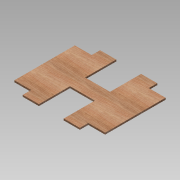
# Autodesk Inventor part: base board
Saved by Autodesk Inventor 2015 (Build 190159000, 159)
## iProperties
Created: 2015-12-17
Part Number: base board
Material: Wood (Birch)
Document SubType Name: Modeling
Designer: Daniel
Density: 0.55 g/cm^3
Appearance: Birch - Natural Polished
Author: Daniel
Autodesk Inventor part; units mm, degrees
ref_plane "YZ Plane" through (0, 0, 0) normal (1, 0, 0) x (0, 1, 0)
ref_plane "XZ Plane" through (0, 0, 0) normal (0, 1, 0) x (-1, 0, 0)
ref_plane "XY Plane" through (0, 0, 0) normal (0, 0, 1) x (1, 0, 0)
sketch "Sketch1" plane through (0, 0, 0) normal (0, 1, 0) x (-1, 0, 0)
  line L0 (0, 0) -> (685.8, 0)
  line L1 (685.8, 0) -> (685.8, -584.2)
  line L2 (685.8, -584.2) -> (0, -584.2)
  line L3 (0, -584.2) -> (0, 0)
  dimension "d0" = 685.8
  dimension "d1" = 584.2
  constraints: 8 end point, 2 parallel, 1 horizontal, 1 perpendicular
  measures "d0" distance of L0.start L0.end
  measures "d1" distance of L2.end L0.start
extrude "Extrusion1" add sketch "Sketch1" along normal blind 12.7
sketch "Sketch2" plane through (0, 12.7, 0) normal (0, 1, 0) x (1, 0, 0)
  line L0 (-436.88, 0) -> (-248.92, 0)
  line L1 (-248.92, 0) -> (-248.92, 234.95)
  line L2 (-248.92, 234.95) -> (-436.88, 234.95)
  line L3 (-436.88, 234.95) -> (-436.88, 0)
  line L4 (0, 584.2) -> (-685.8, 584.2) projected
  line L5 (-436.88, 584.2) -> (-248.92, 584.2)
  line L6 (-248.92, 584.2) -> (-248.92, 349.25)
  line L7 (-248.92, 349.25) -> (-436.88, 349.25)
  line L8 (-436.88, 349.25) -> (-436.88, 584.2)
  line L9 (-685.8, 0) -> (0, 0) projected
  line L10 (-436.88, 349.25) -> (-436.88, 234.95) construction
  line L11 (-685.8, 584.2) -> (-685.8, 0) construction
  point P0 (-342.9, 0)
  point P1 (-342.9, 0)
  point P2 (-342.9, 0)
  point P3 (-342.9, 584.2)
  point P4 (-342.9, 584.2)
  point P5 (-436.88, 292.1)
  point P6 (-685.8, 292.1)
  dimension "d4" = 187.96
  dimension "d6" = 187.96
  dimension "d10" = 114.3
  constraints: 18 end point, 7 midpoint, 4 parallel, 3 coincident, 2 horizontal, 2 perpendicular, 1 horizontal alignment, 1 point on line
  measures "d4" distance of L2.end L1.end
  measures "d6" distance of L6.end L7.end
  measures "d10" distance between parallel lines of L2 L7
extrude "Extrusion2" cut sketch "Sketch2" against normal through all
sketch "Sketch3" plane through (0, 12.7, 0) normal (0, 1, 0) x (1, 0, 0)
  line L0 (0, 0) -> (0, 584.2) projected
  line L1 (0, 0) -> (-127, 0)
  line L2 (-127, 0) -> (-127, 63.5)
  line L3 (-127, 63.5) -> (0, 63.5)
  line L4 (0, 63.5) -> (0, 0)
  line L5 (0, 584.2) -> (-127, 584.2)
  line L6 (-127, 584.2) -> (-127, 520.7)
  line L7 (-127, 520.7) -> (0, 520.7)
  line L8 (0, 520.7) -> (0, 584.2)
  line L9 (-685.8, 584.2) -> (-558.8, 584.2)
  line L10 (-558.8, 584.2) -> (-558.8, 520.7)
  line L11 (-558.8, 520.7) -> (-685.8, 520.7)
  line L12 (-685.8, 520.7) -> (-685.8, 584.2)
  line L13 (-685.8, 0) -> (-558.8, 0)
  line L14 (-558.8, 0) -> (-558.8, 63.5)
  line L15 (-558.8, 63.5) -> (-685.8, 63.5)
  line L16 (-685.8, 63.5) -> (-685.8, 0)
  dimension "d11" = 127
  dimension "d12" = 63.5
  dimension "d13" = 127
  dimension "d14" = 63.5
  dimension "d15" = 127
  dimension "d16" = 63.5
  dimension "d17" = 127
  dimension "d18" = 63.5
  constraints: 32 end point, 8 parallel, 4 horizontal, 4 perpendicular
  measures "d11" distance of L2.end L3.end
  measures "d12" distance of L1.end L2.end
  measures "d13" distance of L7.end L6.end
  measures "d14" distance of L6.end L5.end
  measures "d15" distance of L10.end L11.end
  measures "d16" distance of L9.end L10.end
  measures "d17" distance of L15.end L14.end
  measures "d18" distance of L14.end L13.end
extrude "Extrusion3" cut sketch "Sketch3" against normal through all
body "Solid1"
